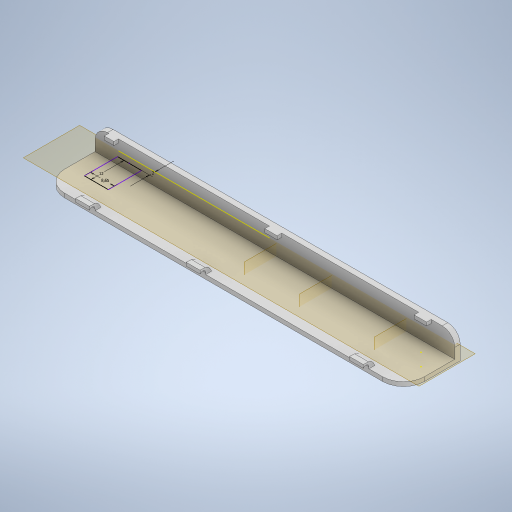
# Autodesk Inventor part: k400+ крышка
Saved by Autodesk Inventor 2024.2 (Build 282272000, 272)
## iProperties
Created: 2025-12-05
Part Number: k400+ крышка
Material: Типовые
Document SubType Name: Modeling
Designer: Zakhar
Density: 1 g/cm^3
Appearance: По умолчанию
Author: Zakhar
Autodesk Inventor part; units mm, degrees
ref_plane "YZ Plane" through (0, 0, 0) normal (1, 0, 0) x (0, 1, 0)
ref_plane "XZ Plane" through (0, 0, 0) normal (0, 1, 0) x (-1, 0, 0)
ref_plane "XY Plane" through (0, 0, 0) normal (0, 0, 1) x (1, 0, 0)
sketch "Эскиз1" plane through (0, 0, 0) normal (0, 1, 0) x (-1, 0, 0)
  line L0 (118.7568, 10.0335) -> (3.7568, 10.0335)
  line L1 (-3.7432, 2.5335) -> (-3.7432, -10.4665)
  line L2 (-3.7432, -10.4665) -> (126.2568, -10.4665)
  line L3 (126.2568, -10.4665) -> (126.2568, 2.5335)
  arc A0 (3.7568, 10.0335) -> (-3.7432, 2.5335) centre (3.7568, 2.5335) ccw
  arc A1 (126.2568, 2.5335) -> (118.7568, 10.0335) centre (118.7568, 2.5335) ccw
  point P0 (0, 0)
  point P1 (-3.7432, 10.0335)
  dimension "d0" = 20.5
  dimension "d1" = 130
  dimension "d2" = 7.5
  dimension "d3" = 7.5
  constraints: 8 end point, 4 point on circle, 4 tangent, 2 centre point, 2 parallel, 2 point on line, 1 horizontal, 1 perpendicular
  measures "d0" distance of point (-3.743, 10.033) L1.end
  measures "d1" distance of L1.end L2.end
  measures "d2" radius of A0
  measures "d3" radius of A1
extrude "Выдавливание1" add sketch "Эскиз1" along normal blind 1.5
sketch "Эскиз2" plane through (0, 1.5, 0) normal (0, 1, 0) x (1, 0, 0)
  line L0 (3.7432, -2.5335) -> (3.7432, 10.4665) projected
  line L1 (-126.2568, 10.4665) -> (-126.2568, -2.5335) projected
  line L2 (3.7432, 10.4665) -> (-126.2568, 10.4665)
  line L3 (-126.2568, 10.4665) -> (-126.2568, 8.4665)
  line L4 (-126.2568, 8.4665) -> (3.7432, 8.4665)
  line L5 (3.7432, 8.4665) -> (3.7432, 10.4665)
  point P0 (0, 0)
  point P1 (3.7432, 8.4665)
  dimension "d6" = 2
  constraints: 8 end point, 2 parallel, 1 horizontal, 1 perpendicular, 1 point on line
  measures "d6" distance between parallel lines of L2 L4
extrude "Выдавливание2" add sketch "Эскиз2" along normal blind 8.2
fillet "Сопряжение1" radius 4.5 1 edges at (3.7432, 9.7, -9.4665)
fillet "Сопряжение2" radius 4.5 1 edges at (-126.2568, 9.7, -9.4665)
sketch "Эскиз3" plane through (-126.2568, 1.5, -8.4665) normal (0, 0, 1) x (1, 0, 0)
  line L0 (125.5, 8.2) -> (4.5, 8.2) projected
  line L1 (117, 8.2) -> (121.5, 8.2)
  line L2 (121.5, 8.2) -> (121.5, 6.95)
  line L3 (121.5, 6.95) -> (117, 6.95)
  line L4 (117, 6.95) -> (117, 8.2)
  line L5 (130, 0) -> (130, 3.7) projected
  line L6 (63, 8.2) -> (67.5, 8.2)
  line L7 (67.5, 8.2) -> (67.5, 6.95)
  line L8 (67.5, 6.95) -> (63, 6.95)
  line L9 (63, 6.95) -> (63, 8.2)
  line L10 (5, 8.2) -> (8.5, 8.2)
  line L11 (8.5, 8.2) -> (8.5, 6.95)
  line L12 (8.5, 6.95) -> (5, 6.95)
  line L13 (5, 6.95) -> (5, 8.2)
  point P0 (126.2568, -1.5)
  point P1 (121.5, 7.575)
  point P2 (63, 7.575)
  point P3 (67.5, 7.575)
  point P4 (8.5, 8.2)
  dimension "d11" = 8.5
  dimension "d12" = 4.5
  dimension "d13" = 1.25
  dimension "d14" = 58.5
  dimension "d15" = 4.5
  dimension "d16" = 1.25
  dimension "d17" = 62.5
  dimension "d18" = 3.5
  dimension "d19" = 1.25
  constraints: 24 end point, 6 parallel, 3 horizontal, 3 midpoint, 3 perpendicular, 2 collinear, 1 point on line
  measures "d11" distance from line of L5 point (121.5, 7.575)
  measures "d12" distance of L2.end L3.end
  measures "d13" distance of L3.end L1.start
  measures "d14" distance of point (63, 7.575) point (121.5, 7.575)
  measures "d15" distance of L7.end L8.end
  measures "d16" distance of L6.end L7.end
  measures "d17" distance from line of L13 point (67.5, 7.575)
  measures "d18" distance of L11.end L12.end
  measures "d19" distance of L10.end L11.end
extrude "Выдавливание3" add sketch "Эскиз3" along normal blind 1.65
ref_plane "РабПлоскость1" through (-13.7568, 0, 2.5335) normal (1, 0, 0) x (0, 0, -1)
sketch "Эскиз4" plane through (-13.7568, 0, 2.5335) normal (1, 0, 0) x (0, 0, -1)
  line L0 (-9.5515, 3.8793) -> (-9.5515, 2.1493)
  line L1 (-9.5515, 3.8793) -> (-7.6452, 3.758)
  line L2 (-6.0216, 2.729) -> (-5.3427, 1.5)
  line L3 (-7.5, 1.5) -> (-7.5, 3.23)
  arc A0 (-6.0216, 2.729) -> (-7.6452, 3.758) centre (-7.7722, 1.762) ccw
  line L4 (-8.5983, 0.5037) -> (-8.5983, 3.23) construction
  line L5 (-9.6967, 1.602) -> (-9.6967, 2.1317)
  line L6 (-7.5, 2.1317) -> (-7.5, 1.602)
  arc A1 (-9.6967, 1.602) -> (-7.5, 1.602) centre (-8.5983, 1.602) ccw
  arc A2 (-7.5, 2.1317) -> (-9.6967, 2.1317) centre (-8.5983, 2.1317) ccw
  line L7 (0, 1.5) -> (-7.5, 1.5) projected
  line L8 (-5.3427, 1.5) -> (-7.5, 1.5)
  point P0 (2.5335, 0)
  point P1 (-6.5515, 3.6883)
  point P2 (-8.5983, 1.8668)
  point P3 (-9.5515, 2.6775)
  dimension "d23" = 1.73
  dimension "d24" = 3
  dimension "d25" = 2.5
  dimension "d26" = 1.73
  dimension "d27" = 2
  constraints: 18 end point, 8 point on circle, 6 tangent, 4 point on line, 3 centre point, 3 vertical, 1 collinear, 1 midpoint, 1 parallel
  measures "d23" distance of L0.start L0.end
  measures "d24" horizontal distance of L0.start point (-6.551, 3.688)
  measures "d25" distance of point (-6.551, 3.688) L2.end
  measures "d26" distance of L3.start L3.end
  measures "d27" radius of A0
extrude "Выдавливание4" add sketch "Эскиз4" along normal blind 5 contours L1 A0 L2 L7 L3 A2 L0
ref_plane "РабПлоскость2" through (-40.7568, 0, 2.5335) normal (1, 0, 0) x (0, 0, -1)
mirror "Зеркальное отражение1" about plane through (-40.7568, 0, 2.5335) normal (1, 0, 0) of "Выдавливание4"
ref_plane "РабПлоскость3" through (-60.7568, 0, 2.5335) normal (1, 0, 0) x (0, 0, -1)
mirror "Зеркальное отражение2" about plane through (-60.7568, 0, 2.5335) normal (1, 0, 0) of "Выдавливание4"
sketch "Эскиз5" plane through (0, 1.5, 0) normal (0, 1, 0) x (1, 0, 0)
  point P0 (0, 0)
ref_plane "РабПлоскость4" through (0, 6, 0) normal (0, 1, 0) x (1, 0, 0)
sketch "Эскиз6" plane through (0, 6, 0) normal (0, 1, 0) x (1, 0, 0)
  line L0 (-107.513, 6.4665) -> (-116.163, 6.4665)
  line L1 (-116.163, 6.4665) -> (-116.163, -5.5335)
  line L2 (-116.163, -5.5335) -> (-107.513, -5.5335)
  line L3 (-107.513, -5.5335) -> (-107.513, 6.4665)
  line L4 (-117.7568, 8.4665) -> (-63.2568, 8.4665) projected
  point P0 (0, 0)
  point P1 (-111.838, 6.4665)
  dimension "d33" = 12
  dimension "d34" = 8.65
  dimension "d35" = 2
  constraints: 8 end point, 2 parallel, 1 horizontal, 1 midpoint, 1 perpendicular
  measures "d33" distance of L0.end L1.end
  measures "d34" distance of L1.end L2.end
  measures "d35" distance from line of L4 point (-111.838, 6.467)
